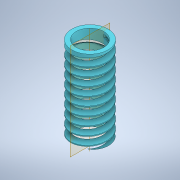
# Autodesk Inventor part: outerShell
Saved by Autodesk Inventor 2021.1 (Build 251245000, 245)
## iProperties
Created: 2020-08-16
Part Number: outerShell
Material: Generic
Document SubType Name: Modeling
Designer: robst
Density: 1 g/cm^3
Appearance: Cadet Blue
Author: robst
Autodesk Inventor part; units mm, degrees
ref_plane "XZ Plane" through (0, 0, 0) normal (0, 1, 0) x (-1, 0, 0)
ref_plane "XY Plane" through (0, 0, 0) normal (0, 0, 1) x (1, 0, 0)
sketch "Sketch1" plane through (0, 0, 0) normal (0, 1, 0) x (-1, 0, 0)
  circle A0 centre (0, 0) radius 26.9875
  circle A1 centre (0, 0) radius 20.6375
  dimension "d0" = 53.975
  dimension "d10" = 41.275
  constraints: 2 centre point, 2 coincident
  measures "d0" diameter of A0
  measures "d10" diameter of A1
extrude "Extrusion2" add sketch "Sketch1" along normal blind 127
sketch "Sketch3" plane through (0, 0, 0) normal (1, 0, 0) x (0, 1, 0)
  line L0 (0, -26.9875) -> (127, -26.9875) projected
  line L1 (127, -26.9875) -> (127, 26.9875) projected
  line L2 (127, -26.9875) -> (121.3198, -17.149)
  line L3 (121.3198, -17.149) -> (115.6395, -26.9875)
  point P0 (0, 0)
  dimension "d13" = 60
  constraints: 4 end point, 1 equal length, 1 point on line
  measures "d13" angle of L3 L2
coil "Coil1" sketch "Sketch3" operation cut axis through (0, -10, 0) along (0, -1, 0) pitch 12.7 turns 10 hand right
body "Solid2"
